Autodesk Inventor part; units mm, degrees
(part 2 of 2)
sketch "스케치26" plane through (0, 0, 0) normal (-1, 0, 0) x (0, 0, 1)
  line L0 (-264, 75.2541) -> (-263.9, 75.2268) projected
  line L1 (-264, 75.2541) -> (-264, 75.2541) projected
  line L2 (-263.9, 75.2268) -> (-264, 75.2541) projected
  line L3 (-263.9, 75.2268) -> (-263.9, 75.2268) projected
  line L4 (-270, 72.5) -> (-270, 75.5) projected
  line L5 (-270, 62.75) -> (-270, 65.25) projected
  line L6 (-264, 65.25) -> (-264, 62.75) projected
  line L7 (-270, 62.75) -> (-270, 65.25) projected
  line L8 (-273.1938, 25.5) -> (-273.1938, 25.5) projected
  line L9 (-273.1938, 25.5) -> (-273.1938, 25.5) projected
  line L10 (-274.5779, 28.5) -> (-274.5779, 28.5) projected
  line L11 (-274.5779, 28.5) -> (-274.5779, 28.5) projected
  line L12 (-278.156, 29.1645) -> (-276.3882, 30.9323) projected
  line L13 (-281.3379, 21.7399) -> (-283.1057, 19.9722) projected
  line L14 (-285.227, 22.0935) -> (-283.4593, 23.8612) projected
  line L15 (-298.9775, 12.1374) -> (-296.8124, 13.3874) projected
  line L16 (-293.8124, 8.1912) -> (-295.9775, 6.9412) projected
  line L17 (-298.9775, 12.1374) -> (-296.8124, 13.3874) projected
  line L18 (-305.8122, 6.1) -> (-305.8122, 6.1) projected
  line L19 (-305.8122, 6.1) -> (-305.8122, 6.1) projected
  line L20 (-304.5877, 1.8546) -> (-302.4226, 3.1046) projected
  line L21 (-307.6377, 7.1374) -> (-305.4726, 8.3874) projected
  line L22 (-305.8122, 6.1) -> (-305.8122, 6.1) projected
  line L23 (-305.8122, 6.1) -> (-305.8122, 6.1) projected
  line L24 (-304.75, 0) -> (-307.25, 0) projected
  line L25 (-234.25, 6) -> (-231.75, 6) projected
  line L26 (-231.75, 0) -> (-234.25, 0) projected
  line L27 (-161.25, 6) -> (-158.75, 6) projected
  line L28 (-158.75, 0) -> (-161.25, 0) projected
  line L29 (-88.25, 6) -> (-85.75, 6) projected
  line L30 (-85.75, 0) -> (-88.25, 0) projected
  line L31 (-14.1878, 6.1) -> (-14.1878, 6.1) projected
  line L32 (-14.1878, 6.1) -> (-14.1878, 6.1) projected
  line L33 (-12.75, 0) -> (-15.25, 0) projected
  line L34 (-14.1878, 6.1) -> (-14.1878, 6.1) projected
  line L35 (-14.1878, 6.1) -> (-14.1878, 6.1) projected
  line L36 (-17.5774, 3.1046) -> (-15.4123, 1.8546) projected
  line L37 (-14.5274, 8.3874) -> (-12.3623, 7.1374) projected
  line L38 (-24.0225, 6.9412) -> (-26.1876, 8.1912) projected
  line L39 (-23.1876, 13.3874) -> (-21.0225, 12.1374) projected
  line L40 (-36.9086, 19.9864) -> (-38.6763, 21.7542) projected
  line L41 (-36.555, 23.8755) -> (-34.7873, 22.1078) projected
  line L42 (-46.8062, 25.5) -> (-46.8062, 25.5) projected
  line L43 (-46.8062, 25.5) -> (-46.8062, 25.5) projected
  line L44 (-45.4221, 28.5) -> (-45.4221, 28.5) projected
  line L45 (-45.4221, 28.5) -> (-45.4221, 28.5) projected
  line L46 (-43.6261, 30.9466) -> (-41.8583, 29.1788) projected
  line L47 (-56, 62.5) -> (-56, 65.5) projected
  line L48 (-50, 65.5) -> (-50, 62.5) projected
  line L49 (-56, 75.2541) -> (-56.1, 75.2268) projected
  line L50 (-56, 75.2541) -> (-56, 75.2541) projected
  line L51 (-56.1, 75.2268) -> (-56, 75.2541) projected
  line L52 (-56.1, 75.2268) -> (-56.1, 75.2268) projected
  line L53 (-50, 75.5) -> (-50, 72.5) projected
  arc A0 (-270, 73.3386) -> (-270, 74.6614) centre (-270.75, 74) ccw
  arc A1 (-270, 63.3386) -> (-270, 64.6614) centre (-270.75, 64) ccw
  arc A2 (-277.7398, 29.5807) -> (-276.8044, 30.5161) centre (-277.8024, 30.5788) ccw
  arc A3 (-284.8109, 22.5097) -> (-283.8754, 23.4451) centre (-284.8735, 23.5077) ccw
  arc A4 (-298.4677, 12.4317) -> (-297.3221, 13.0931) centre (-298.2699, 13.4119) ccw
  arc A5 (-307.128, 7.4317) -> (-305.9824, 8.0931) centre (-306.9302, 8.4119) ccw
  arc A6 (-305.3386, 0) -> (-306.6614, 0) centre (-306, -0.75) ccw
  arc A7 (-232.3386, 0) -> (-233.6614, 0) centre (-233, -0.75) ccw
  arc A8 (-159.3386, 0) -> (-160.6614, 0) centre (-160, -0.75) ccw
  arc A9 (-86.3386, 0) -> (-87.6614, 0) centre (-87, -0.75) ccw
  arc A10 (-13.3386, 0) -> (-14.6614, 0) centre (-14, -0.75) ccw
  arc A11 (-14.0176, 8.0931) -> (-12.872, 7.4317) centre (-13.0698, 8.4119) ccw
  arc A12 (-22.6779, 13.0931) -> (-21.5323, 12.4317) centre (-21.7301, 13.4119) ccw
  arc A13 (-36.1388, 23.4594) -> (-35.2034, 22.5239) centre (-35.1408, 23.522) ccw
  arc A14 (-43.2099, 30.5304) -> (-42.2745, 29.595) centre (-42.2119, 30.593) ccw
  arc A15 (-50, 64.6614) -> (-50, 63.3386) centre (-49.25, 64) ccw
  arc A16 (-50, 74.6614) -> (-50, 73.3386) centre (-49.25, 74) ccw
  point P0 (0, 0)
  dimension "d279" = 2
  dimension "d280" = 2
  dimension "d281" = 2
  dimension "d282" = 2
  dimension "d283" = 2
  dimension "d284" = 2
  dimension "d285" = 2
  dimension "d286" = 2
  dimension "d287" = 2
  dimension "d288" = 2
  dimension "d289" = 2
  dimension "d290" = 2
  dimension "d291" = 2
  dimension "d292" = 2
  dimension "d293" = 2
  dimension "d294" = 2
  dimension "d295" = 2
  dimension "d296" = 0.75
  dimension "d297" = 0.75
  dimension "d298" = 0.75
  dimension "d299" = 0.75
  dimension "d300" = 0.75
  dimension "d301" = 0.75
  dimension "d302" = 0.75
  dimension "d303" = 0.75
  dimension "d304" = 0.75
  dimension "d305" = 0.75
  dimension "d306" = 0.75
  dimension "d307" = 0.75
  dimension "d308" = 0.75
  dimension "d309" = 0.75
  dimension "d310" = 0.75
  dimension "d311" = 0.75
  dimension "d312" = 0.75
  constraints: 34 point on circle, 34 point on line, 17 centre point
  measures "d279" diameter of A0
  measures "d280" diameter of A1
  measures "d281" diameter of A2
  measures "d282" diameter of A3
  measures "d283" diameter of A4
  measures "d284" diameter of A5
  measures "d285" diameter of A6
  measures "d286" diameter of A7
  measures "d287" diameter of A8
  measures "d288" diameter of A9
  measures "d289" diameter of A10
  measures "d290" diameter of A11
  measures "d291" diameter of A12
  measures "d292" diameter of A13
  measures "d293" diameter of A14
  measures "d294" diameter of A15
  measures "d295" diameter of A16
  measures "d296" distance from line of L53 A16.centre
  measures "d297" distance from line of L48 A15.centre
  measures "d298" distance from line of L46 A14.centre
  measures "d299" distance from line of L41 A13.centre
  measures "d300" distance from line of L39 A12.centre
  measures "d301" distance from line of L37 A11.centre
  measures "d302" distance from line of L33 A10.centre
  measures "d303" distance from line of L30 A9.centre
  measures "d304" distance from line of L28 A8.centre
  measures "d305" distance from line of L26 A7.centre
  measures "d306" distance from line of L24 A6.centre
  measures "d307" distance from line of L21 A5.centre
  measures "d308" distance from line of L15 A4.centre
  measures "d309" distance from line of L14 A3.centre
  measures "d310" distance from line of L12 A2.centre
  measures "d311" distance from line of L5 A1.centre
  measures "d312" distance from line of L4 A0.centre
extrude "돌출29" cut sketch "스케치26" against normal blind 8
